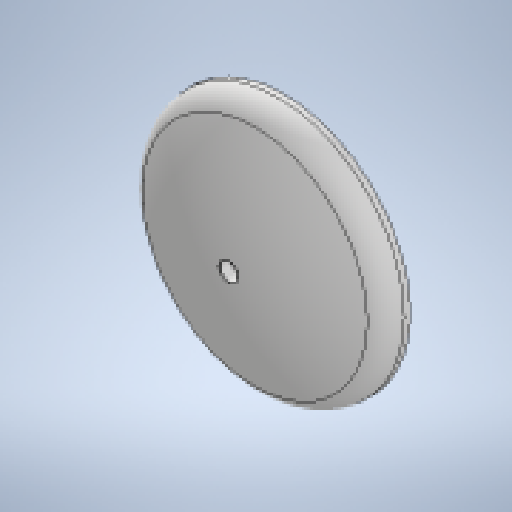
# Autodesk Inventor part: Фильтр напорный угольный 30 куб час
Saved by Autodesk Inventor 2025.1 (Build 291241020, 241B)
## iProperties
Created: 2024-12-11
Part Number: Фильтр напорный угольный 30 куб час
Material: Generic
Document SubType Name: Modeling
Designer: user
Density: 1 g/cm^3
Appearance: Default
Author: user
Autodesk Inventor part; units mm, degrees
ref_plane "YZ Plane" through (0, 0, 0) normal (1, 0, 0) x (0, 1, 0)
ref_plane "XY Plane" through (0, 0, 0) normal (0, 0, 1) x (1, 0, 0)
sketch "Sketch1" plane through (0, 0, 0) normal (0, 0, 1) x (1, 0, 0)
  line L0 (-977.7778, 659.2259) -> (977.7778, 659.2259) construction
  arc A0 (-977.7778, 659.2259) -> (0, 430) centre (0, 2630) ccw construction
  line L1 (-1100, 856.3033) -> (1100, 856.3033) construction
  arc A1 (-1100, 856.3033) -> (-977.7778, 659.2259) centre (-880, 856.3033) ccw construction
  arc A2 (977.7778, 659.2259) -> (1100, 856.3033) centre (880, 856.3033) ccw
  line L2 (-1100, 856.3033) -> (-1100, 909.3033)
  line L3 (1100, 856.3033) -> (1100, 909.3033)
  line L4 (-1100, 909.3033) -> (0, 909.3033) construction
  line L5 (0, 909.3033) -> (0, 0)
  arc A3 (0, 430) -> (977.7778, 659.2259) centre (0, 2630) ccw
  line L6 (0, 909.3033) -> (1100, 909.3033)
  dimension "d0" = 2200
  dimension "d1" = 220
  dimension "d2" = 53
  dimension "d3" = 2200
  dimension "d7_from_floor" = 430
  constraints: 14 end point, 8 point on circle, 4 centre point, 4 tangent, 3 horizontal, 3 vertical, 2 equal length, 1 equal radius, 1 point on line, 1 vertical alignment
  measures "d0" radius of A0
  measures "d1" radius of A1
  measures "d2" distance of L1.start L2.end
  measures "d3" distance of L1.start L1.end
  measures "d7_from_floor" distance of L5.end A0.end
revolve "Revolution1" add sketch "Sketch1" angle 360 about axis through (0, 909.3033, 0) along (0, -1, 0)
shell "Shell1" thickness 8 removed faces 1 at (-192.246, 909.3033, 312.2274)
sketch "Sketch2" plane through (0, 0, 0) normal (0, 1, 0) x (-1, 0, 0)
  circle A0 centre (0, 0) radius 81.15
  dimension "d10" = 162.3
  constraints: 1 centre point, 1 coincident
  measures "d10" diameter of A0
extrude "Extrusion1" cut sketch "Sketch2" along normal through all
ref_plane "Work Plane2" through (0, 430, 0) normal (0, 1, 0) x (-1, 0, 0)
sketch "Sketch3" plane through (0, 430, 0) normal (0, 1, 0) x (-1, 0, 0)
  circle A0 centre (0, 0) radius 81.15 projected
  circle A1 centre (0, 0) radius 84.15
  dimension "d14" = 168.3
  constraints: 1 centre point, 1 coincident
  measures "d14" diameter of A1
extrude "Extrusion2" add sketch "Sketch3" along normal blind 120
sketch "Sketch4" plane through (0, 550, 0) normal (0, 1, 0) x (1, 0, 0)
  circle A0 centre (0, 0) radius 81.15 projected
  circle A1 centre (0, 0) radius 140
  dimension "d17" = 280
  constraints: 1 centre point, 1 coincident
  measures "d17" diameter of A1
extrude "Extrusion3" add sketch "Sketch4" against normal blind 22
sketch "Sketch5" plane through (0, 550, 0) normal (0, 1, 0) x (1, 0, 0)
  circle A0 centre (0, 0) radius 140 construction
  circle A1 centre (0, 0) radius 81.15 construction
  circle A2 centre (0, 0) radius 120 construction
  circle A3 centre (-120, 0) radius 10.5
  line L0 (-120, 0) -> (0, 0)
  line L1 (0, 0) -> (-81.15, 0)
  dimension "d20" = 240
  dimension "d21" = 21
  dimension "d22" = 0
  constraints: 4 end point, 2 horizontal alignment, 1 centre point, 1 coincident, 1 horizontal, 3 other
  measures "d21" diameter of A3
  measures "d22" distance between parallel lines of L1 L0
extrude "Extrusion4" cut sketch "Sketch5" against normal blind 22
pattern_circular "Circular Pattern1" count 8 over 360 about axis through (0, 0, 0) along (0, 1, 0) of "Extrusion4"
equation "\"d23\" = d18"
equation "\"d18\" = 22"
body "Solid1"
